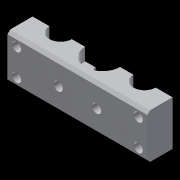
# Autodesk Inventor part: AXBv2
Saved by Autodesk Inventor 2016 (Build 200138000, 138)
## iProperties
Created: 2014-12-25
Part Number: AXBv2
Material: PC/ABS Plastic
Document SubType Name: Modeling
Designer: Jose
Density: 0.357273 g/cm^3
Appearance: Smooth - White
Mass: 15.468 g
Surface Area: 130.353 cm^2
Volume: 43.2946 cm^3
Author: Jose
Autodesk Inventor part; units mm, degrees
ref_plane "YZ Plane" through (0, 0, 0) normal (1, 0, 0) x (0, 1, 0)
ref_plane "XZ Plane" through (0, 0, 0) normal (0, 1, 0) x (-1, 0, 0)
ref_plane "XY Plane" through (0, 0, 0) normal (0, 0, 1) x (1, 0, 0)
sketch "Sketch1" plane through (0, 0, 0) normal (0, 1, 0) x (-1, 0, 0)
  line L0 (-50, 16) -> (50, 16)
  line L1 (50, 16) -> (50, -16)
  line L2 (50, -16) -> (-50, -16)
  line L3 (-50, -16) -> (-50, 16)
  point P0 (0, 0)
  point P1 (-50, 0)
  point P2 (0, 16)
  dimension "d0" = 100
  dimension "d1" = 32
  constraints: 8 end point, 2 midpoint, 2 parallel, 1 horizontal, 1 horizontal alignment, 1 perpendicular, 1 vertical alignment
  measures "d0" distance of L0.start L0.end
  measures "d1" distance of L0.end L1.end
extrude "Extrusion1" add sketch "Sketch1" along normal blind 18
sketch "Sketch7" plane through (50, 0, -16) normal (0, 0, -1) x (-1, 0, 0)
  line L0 (100, 0) -> (0, 0) projected
  line L1 (100, 0) -> (100, 18) projected
  line L2 (0, 18) -> (100, 18) projected
  line L3 (0, 0) -> (0, 18) projected
  circle A0 centre (20, 18) radius 8
  line L4 (100, 18) -> (0, 18) projected
  circle A1 centre (80, 18) radius 8
  line L5 (20, 18) -> (80, 18) construction
  circle A2 centre (50, 18) radius 5
  point P0 (50, 0)
  dimension "d32" = 60
  dimension "d33" = 16
  dimension "d34" = 10
  constraints: 3 centre point, 2 coincident, 2 end point, 2 midpoint, 2 point on line, 1 collinear, 1 equal radius
  measures "d32" distance of L5.end L5.start
  measures "d33" diameter of A0
  measures "d34" diameter of A2
extrude "Extrusion7" cut sketch "Sketch7" against normal through all contours A1 L2 | L2 A1 | A0 L2 | L2 A0 | A2 L2 | L2 A2
sketch "Sketch8" plane through (50, 0, -16) normal (0, 0, -1) x (-1, 0, 0)
  arc A0 (72, 18) -> (88, 18) centre (80, 18) ccw projected
  line L0 (55, 18) -> (72, 18) projected
  arc A1 (45, 18) -> (55, 18) centre (50, 18) ccw projected
  line L1 (28, 18) -> (45, 18) projected
  arc A2 (12, 18) -> (28, 18) centre (20, 18) ccw projected
  line L2 (0, 18) -> (12, 18) projected
  line L3 (0, 0) -> (0, 18) projected
  line L4 (100, 0) -> (0, 0) projected
  line L5 (100, 0) -> (100, 18) projected
  line L6 (88, 18) -> (100, 18) projected
  circle A3 centre (50, 18) radius 12
  point P0 (50, 0)
  dimension "d37" = 24
  constraints: 1 centre point, 1 coincident
  measures "d37" diameter of A3
extrude "Extrusion8" cut sketch "Sketch8" against normal blind 9 contours A3 L1 A1 L0 | L0 A1 L1 A3
sketch "Sketch9" plane through (-50, 0, 16) normal (0, 0, 1) x (1, 0, 0)
  arc A0 (12, 18) -> (28, 18) centre (20, 18) ccw projected
  line L0 (0, 18) -> (12, 18) projected
  line L1 (0, 0) -> (0, 18) projected
  line L2 (100, 0) -> (0, 0) projected
  line L3 (100, 0) -> (100, 18) projected
  line L4 (88, 18) -> (100, 18) projected
  arc A1 (72, 18) -> (88, 18) centre (80, 18) ccw projected
  line L5 (55, 18) -> (72, 18) projected
  arc A2 (45, 18) -> (55, 18) centre (50, 18) ccw projected
  line L6 (28, 18) -> (45, 18) projected
  arc A3 (45, 18) -> (55, 18) centre (50, 18) ccw projected
  circle A4 centre (50, 18) radius 12.5
  point P0 (50, 18)
  dimension "d49" = 25
  constraints: 1 centre point, 1 coincident
  measures "d49" diameter of A4
extrude "Extrusion9" cut sketch "Sketch9" against normal blind 9 contours A4 L5 A2 L6 | L6 A2 L5 A4
sketch "Sketch11" plane through (0, 0, 0) normal (0, -1, 0) x (1, 0, 0)
  circle A0 centre (43.5, -9.5) radius 3
  circle A1 centre (43.5, 9.5) radius 3
  circle A2 centre (13.7, 0) radius 3
  circle A3 centre (-13.7, 0) radius 3
  circle A4 centre (-43.5, -9.5) radius 3
  circle A5 centre (-43.5, 9.5) radius 3
  circle A6 centre (43.5, 9.5) radius 3.2
  circle A7 centre (43.5, -9.5) radius 3.2
  circle A8 centre (13.7, 0) radius 3.2
  circle A9 centre (-13.7, 0) radius 3.2
  circle A10 centre (-43.5, -9.5) radius 3.2
  circle A11 centre (-43.5, 9.5) radius 3.2
  point P0 (0, 0)
  dimension "d50" = 0.2
  constraints: 12 centre point, 5 equal radius, 12 other
  measures "d50" radial gap between concentric circles of A6 A1
extrude "Extrusion10" cut sketch "Sketch11" against normal through all contours A0 | A1 | A2 | A3 | A4 | A5 | A6 | A7 | A8 | A9 | A10 | A11
chamfer "Chamfer3" distance 2 angle 45 2 edges at (0, 0, -16) (0, 0, 16)
body "Solid1"
